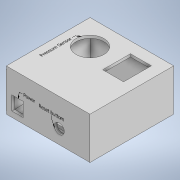
# Autodesk Inventor part: Part3
Saved by Autodesk Inventor 2020 (Build 240168000, 168)
## iProperties
Created: 2019-04-13
Part Number: Part3
Material: Generic
Document SubType Name: Modeling
Designer: cesar
Density: 1 g/cm^3
Appearance: Default
Author: cesar
Autodesk Inventor part; units mm, degrees
ref_plane "YZ Plane" through (0, 0, 0) normal (1, 0, 0) x (0, 1, 0)
ref_plane "XZ Plane" through (0, 0, 0) normal (0, 1, 0) x (-1, 0, 0)
ref_plane "XY Plane" through (0, 0, 0) normal (0, 0, 1) x (1, 0, 0)
sketch "Sketch1" plane through (0, 0, 0) normal (0, 1, 0) x (-1, 0, 0)
  line L0 (59.9595, 0.0507) -> (-0.0405, 0.0507)
  line L1 (-0.0405, 0.0507) -> (-0.0405, -59.9493)
  line L2 (-0.0405, -59.9493) -> (59.9595, -59.9493)
  line L3 (59.9595, -59.9493) -> (59.9595, 0.0507)
  line L4 (54, -52.088) -> (6, -52.088)
  line L5 (6, -52.088) -> (6, -50.088)
  line L6 (6, -50.088) -> (54, -50.088)
  line L7 (54, -50.088) -> (54, -52.088)
  line L8 (54, -46.088) -> (6, -46.088)
  line L9 (6, -46.088) -> (6, -44.088)
  line L10 (6, -44.088) -> (54, -44.088)
  line L11 (54, -44.088) -> (54, -46.088)
  line L12 (54, -40.088) -> (6, -40.088)
  line L13 (6, -40.088) -> (6, -38.088)
  line L14 (6, -38.088) -> (54, -38.088)
  line L15 (54, -38.088) -> (54, -40.088)
  line L16 (54, -34.088) -> (6, -34.088)
  line L17 (6, -34.088) -> (6, -32.088)
  line L18 (6, -32.088) -> (54, -32.088)
  line L19 (54, -32.088) -> (54, -34.088)
  line L20 (54, -28.0372) -> (6, -28.0372)
  line L21 (6, -28.0372) -> (6, -26.088)
  line L22 (6, -26.088) -> (54, -26.088)
  line L23 (54, -26.088) -> (54, -28.0372)
  line L24 (54, -22.088) -> (6, -22.088)
  line L25 (6, -22.088) -> (6, -20.088)
  line L26 (6, -20.088) -> (54, -20.088)
  line L27 (54, -20.088) -> (54, -22.088)
  line L28 (54, -16.088) -> (6, -16.088)
  line L29 (6, -16.088) -> (6, -14.088)
  line L30 (6, -14.088) -> (54, -14.088)
  line L31 (54, -14.088) -> (54, -16.088)
  line L32 (54, -10.088) -> (6, -10.088)
  line L33 (6, -10.088) -> (6, -8.088)
  line L34 (6, -8.088) -> (54, -8.088)
  line L35 (54, -8.088) -> (54, -10.088)
  line L36 (2, -58) -> (58, -58)
  line L37 (58, -58) -> (58, -2)
  line L38 (58, -2) -> (2, -2)
  line L39 (2, -2) -> (2, -58)
  point P0 (0, 0)
  dimension "d0" = 60
  dimension "d1" = 60
  constraints: 80 end point, 19 parallel, 11 perpendicular, 10 horizontal, 6 point on line
  measures "d0" distance of L2.end L0.start
  measures "d1" distance of L0.start L0.end
extrude "Bottom" add sketch "Sketch1" along normal blind 2 contours L3 L2 L1 L0 | L39 L38 L37 L36
sketch "Sketch2" plane through (0, 2, 0) normal (0, 1, 0) x (1, 0, 0)
  line L0 (-59.9595, -0.0507) -> (0.0405, -0.0507) projected
  line L1 (-60, 59.9493) -> (-58, 59.9493)
  line L2 (-58, 59.9493) -> (-58, -0.0507)
  line L3 (-58, -0.0507) -> (-60, -0.0507)
  line L4 (-60, -0.0507) -> (-60, 59.9493)
  line L5 (0.0405, 59.9493) -> (-59.9595, 59.9493) projected
  line L6 (-2, 59.9493) -> (0.0405, 59.9493)
  line L7 (0.0405, 59.9493) -> (0.0405, -0.0507)
  line L8 (0.0405, -0.0507) -> (-2, -0.0507)
  line L9 (-2, -0.0507) -> (-2, 59.9493)
  line L10 (-58, 59.9493) -> (-2, 59.9493)
  line L11 (-2, 59.9493) -> (-2, 58)
  line L12 (-2, 58) -> (-58, 58)
  line L13 (-58, 58) -> (-58, 59.9493)
  line L14 (-58, 2) -> (-2, 2)
  line L15 (-2, 2) -> (-2, -0.0507)
  line L16 (-2, -0.0507) -> (-58, -0.0507)
  line L17 (-58, -0.0507) -> (-58, 2)
  point P0 (-2, 2)
  constraints: 32 end point, 8 parallel, 4 horizontal, 4 perpendicular, 4 point on line
extrude "Walls" add sketch "Sketch2" along normal blind 26 contours L3 L4 L1 L2 L0 | L2 L14 L9 L0 | L9 L5 L7 L0 | L2 L5 L9 L12
sketch "Sketch3" plane through (-59.9595, 0, 0.0507) normal (0, 0, 1) x (1, 0, 0)
  line L0 (4, 4) -> (12, 4)
  line L1 (12, 4) -> (12, 14)
  line L2 (12, 14) -> (4, 14)
  line L3 (4, 14) -> (4, 4)
  line L4 (5.6179, 18.3587) -> (10.1248, 18.3587) construction
  line L5 (10.1248, 18.3587) -> (10.1248, 14.1529) construction
  line L6 (10.1248, 14.1529) -> (5.6179, 14.1529) construction
  line L7 (5.6179, 14.1529) -> (5.6179, 18.3587) construction
  circle A0 centre (38, 10) radius 3.6056
  line L8 (32.7887, 17.939) -> (43.0738, 17.939) construction
  line L9 (43.0738, 17.939) -> (43.0738, 14.8367) construction
  line L10 (43.0738, 14.8367) -> (32.7887, 14.8367) construction
  line L11 (32.7887, 14.8367) -> (32.7887, 17.939) construction
  point P0 (59.9595, 0)
  constraints: 8 end point, 2 parallel, 1 centre point, 1 horizontal, 1 perpendicular, 4 other
extrude "AC/Reset" cut sketch "Sketch3" against normal blind 10
sketch "Sketch4" plane through (0, 28, 0) normal (0, 1, 0) x (1, 0, 0)
  line L0 (0.0405, -0.0507) -> (0.0405, 59.9493) projected
  line L1 (-59.9595, 60) -> (0.0405, 60)
  line L2 (0.0405, 60) -> (0.0405, -0.0507)
  line L3 (0.0405, -0.0507) -> (-59.9595, -0.0507)
  line L4 (-59.9595, -0.0507) -> (-59.9595, 60)
  circle A0 centre (-42, 42) radius 10
  line L5 (-6, 32.088) -> (-54, 32.088) projected
  line L6 (-23, 52) -> (-8, 52)
  line L7 (-8, 52) -> (-8, 32.088)
  line L8 (-8, 32.088) -> (-23, 32.088)
  line L9 (-23, 32.088) -> (-23, 52)
  point P0 (0, 0)
  dimension "d8" = 20
  dimension "d9" = 60
  constraints: 16 end point, 4 parallel, 2 horizontal, 2 perpendicular, 1 centre point, 1 point on line
  measures "d8" diameter of A0
  measures "d9" distance of L1.start L1.end
extrude "Extrusion4" add sketch "Sketch4" along normal blind 2
body "Solid1"
